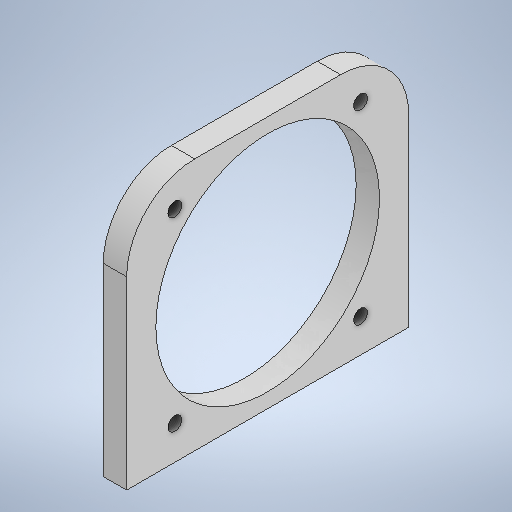
# Autodesk Inventor part: Gear_support
Saved by Autodesk Inventor 2025.2 (Build 292293000, 293)
## iProperties
Created: 2025-02-20
Part Number: Gear_support
Material: Generic
Document SubType Name: Modeling
Designer: Sergio Quintero
Density: 1 g/cm^3
Appearance: Default
Author: Sergio Quintero
Autodesk Inventor part; units mm, degrees
ref_plane "YZ Plane" through (0, 0, 0) normal (1, 0, 0) x (0, 1, 0)
ref_plane "XZ Plane" through (0, 0, 0) normal (0, 1, 0) x (-1, 0, 0)
ref_plane "XY Plane" through (0, 0, 0) normal (0, 0, 1) x (1, 0, 0)
sketch "Sketch1" plane through (0, 0, 0) normal (1, 0, 0) x (0, 1, 0)
  line L0 (-65, -72.5) -> (65, -72.5)
  line L1 (65, -72.5) -> (65, 72.5)
  line L2 (65, 72.5) -> (-65, 72.5)
  line L3 (-65, 72.5) -> (-65, -72.5)
  line L4 (-65, -72.5) -> (65, 72.5) construction
  line L5 (65, -72.5) -> (-65, 72.5) construction
  point P0 (0, 0)
  dimension "d0" = 130
  dimension "d1" = 145
  constraints: 12 end point, 2 midpoint, 2 parallel, 1 horizontal, 1 perpendicular
  measures "d0" distance of L2.end L1.end
  measures "d1" distance of L1.end L0.end
extrude "Extrusion1" add sketch "Sketch1" along normal blind 12
fillet "Fillet1" radius 35 2 edges at (6, 65, 72.5) (6, 65, -72.5)
sketch "Sketch2" plane through (0, -65, -72.5) normal (0, -1, 0) x (1, 0, 0)
  line L0 (0, 145) -> (12, 145) projected
  line L1 (0, 0) -> (12, 0) projected
  line L2 (12, 145) -> (12, 0) projected
  point P0 (0, 72.5)
  point P1 (6, 137.5)
  point P2 (6, 7.5)
  point P3 (6, 145)
  point P4 (6, 0)
  dimension "d5" = 7.5
  dimension "d6" = 7.5
  dimension "d7" = 6
  dimension "d8" = 6
  constraints: 2 midpoint
  measures "d5" distance of point (6, 145) point (6, 137.5)
  measures "d6" distance of point (6, 0) point (6, 7.5)
  measures "d7" distance from line of point (6, 7.5) L2
  measures "d8" distance from line of L2 point (6, 137.5)
hole "Hole1" at (6, -65, 65) at (6, -65, -65) direction (0, 1, 0) diameter 7.134 depth 20.2 tip angle 118 thread size "M8x0.8" class "6H" standard "ISO Metric profile"
sketch "Sketch3" plane through (12, 0, 0) normal (1, 0, 0) x (0, 0, -1)
  circle A0 centre (0, 0) radius 57.5
  dimension "d16" = 115
  constraints: 1 centre point, 1 coincident
  measures "d16" diameter of A0
extrude "Extrusion2" cut sketch "Sketch3" against normal blind 12
sketch "Sketch4" plane through (12, 0, 0) normal (1, 0, 0) x (0, 0, -1)
  circle A0 centre (0, 0) radius 67.5 construction
  line L0 (0, 0) -> (-82.2434, 82.2434) construction
  line L1 (0, 0) -> (116.3098, 0) construction
  point P0 (-47.7297, 47.7297)
  dimension "d19" = 135
  dimension "d20" = 135
  constraints: 4 end point, 1 coincident, 1 equal length, 1 horizontal, 1 point on line, 3 other
  measures "d20" angle of L1 L0
hole "Hole2" at (12, 47.7297, 47.7297) direction (-1, 0, 0) diameter 7.134 depth 20.2 tip angle 118 thread size "M8x0.8" class "6H" standard "ISO Metric profile"
pattern_circular "Circular Pattern1" count 4 over 360 about axis through (-10, 0, 0) along (1, 0, 0) of "Hole2"
body "Solid1"
